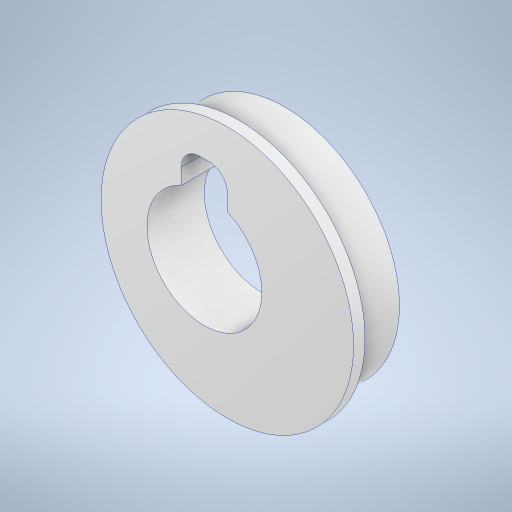
# Autodesk Inventor part: 偏心軸板
Saved by Autodesk Inventor 2024 (Build 280153000, 153)
## iProperties
Created: 2023-05-29
Part Number: 偏心軸板
Material: アルミニウム 6061
Document SubType Name: Modeling
Designer: yuta2
Density: 2.7 g/cm^3
Appearance: アルミニウム - フラット
Author: yuta2
Autodesk Inventor part; units mm, degrees
ref_plane "YZ Plane" through (0, 0, 0) normal (1, 0, 0) x (0, 1, 0)
ref_plane "XZ Plane" through (0, 0, 0) normal (0, 1, 0) x (-1, 0, 0)
ref_plane "XY Plane" through (0, 0, 0) normal (0, 0, 1) x (1, 0, 0)
sketch "スケッチ1" plane through (0, 0, 0) normal (0, 0, 1) x (1, 0, 0)
  circle A0 centre (0, 0) radius 10
  dimension "d0" = 20
  constraints: 1 centre point, 1 coincident
  measures "d0" diameter of A0
extrude "押し出し1" add sketch "スケッチ1" along normal blind 5
sketch "スケッチ2" plane through (0, 0, 5) normal (0, 0, 1) x (1, 0, 0)
  circle A0 centre (0, 0) radius 10 projected
  circle A1 centre (0, 0) radius 11
  circle A2 centre (0, 0) radius 10 projected
  dimension "d3" = 22
  constraints: 1 centre point, 1 coincident
  measures "d3" diameter of A1
extrude "押し出し2" add sketch "スケッチ2" against normal blind 1
sketch "スケッチ3" plane through (0, 0, 0) normal (0, 0, -1) x (-1, 0, 0)
  point P0 (0, 0)
  point P1 (2, 0)
  dimension "d6" = 2
  constraints: 1 horizontal alignment
  measures "d6" distance of point (0, 0) point (2, 0)
hole "穴1" at (-2, 0, 0) direction (0, 0, 1) diameter 10 end through all
sketch "スケッチ4" plane through (0, 0, 0) normal (0, 0, -1) x (-1, 0, 0)
  circle A0 centre (2, 0) radius 5 projected
  line L0 (0, 4.5826) -> (4, 4.5826)
  line L1 (4, 4.5826) -> (4, 5.9826)
  line L2 (2.4, 7.5826) -> (1.6, 7.5826)
  line L3 (0, 5.9826) -> (0, 4.5826)
  arc A1 (1.6, 7.5826) -> (0, 5.9826) centre (1.6, 5.9826) ccw
  arc A2 (4, 5.9826) -> (2.4, 7.5826) centre (2.4, 5.9826) ccw
  point P0 (0, 0)
  point P1 (4, 7.5826)
  point P2 (0, 7.5826)
  dimension "d14" = 4
  dimension "d15" = 3
  dimension "d18" = 1.6
  dimension "d19" = 1.6
  constraints: 8 end point, 6 point on circle, 4 point on line, 4 tangent, 2 centre point, 2 parallel, 1 horizontal, 1 perpendicular
  measures "d14" distance of point (4, 7.583) point (0, 7.583)
  measures "d15" distance of point (0, 7.583) L0.start
  measures "d18" radius of A1
  measures "d19" radius of A2
extrude "押し出し3" cut sketch "スケッチ4" against normal through all contours L0 A0 | A0 L3 A1 L2 A2 L1 picked at (1.6595, 4.6866)
equation "\"d6\" = r"
equation "\"r\" = 2"
